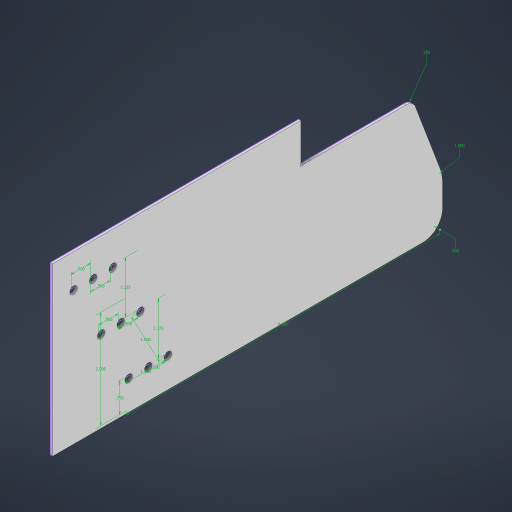
# Autodesk Inventor part: dtplate
Saved by Autodesk Inventor 2024 (Build 280153000, 153)
## iProperties
Created: 2023-11-04
Part Number: dtplate
Material: Generic
Document SubType Name: Modeling
Designer: macbook
Density: 1 g/cm^3
Appearance: Default
Author: macbook
Autodesk Inventor part; units mm, degrees
ref_plane "YZ Plane" through (0, 0, 0) normal (1, 0, 0) x (0, 1, 0)
ref_plane "XZ Plane" through (0, 0, 0) normal (0, 1, 0) x (-1, 0, 0)
ref_plane "XY Plane" through (0, 0, 0) normal (0, 0, 1) x (1, 0, 0)
sketch "Sketch1" plane through (0, 0, 0) normal (1, 0, 0) x (0, 1, 0)
  line L0 (0, -19.05) -> (0, -190.5)
  line L1 (12.7, -203.2) -> (27.1441, -203.2)
  arc A0 (82.55, -117.475) -> (63.5, -95.25) centre (61.8713, -115.9228) ccw
  line L2 (82.55, -117.475) -> (82.55, -179.7494)
  arc A1 (0, -190.5) -> (12.7, -203.2) centre (12.7, -190.5) ccw
  arc A2 (78.4296, -185.6951) -> (82.55, -179.7494) centre (76.2, -179.7494) ccw
  arc A3 (27.1441, -203.2) -> (36.0626, -201.5828) centre (27.1441, -177.8) ccw
  line L3 (78.4296, -185.6951) -> (36.0626, -201.5828)
  line L4 (19.05, 0) -> (19.05, -25.4)
  line L5 (19.05, -25.4) -> (19.05, -12.7)
  line L6 (19.05, -25.4) -> (57.15, -25.4) construction
  line L7 (19.05, -25.4) -> (52.705, -25.4)
  line L8 (52.705, -25.4) -> (52.705, -7.5157)
  line L9 (19.05, -25.4) -> (52.705, -7.5408)
  line L10 (0, -19.05) -> (0, 49.2218)
  line L11 (0, 49.2218) -> (63.5, 49.2218)
  line L12 (52.705, -7.5408) -> (52.705, 5.1592)
  line L13 (52.705, 5.1592) -> (52.705, 17.8592)
  line L14 (52.705, -7.5408) -> (86.36, -7.5408)
  line L15 (52.705, -7.5408) -> (86.36, 10.3184)
  line L16 (86.36, 10.3184) -> (86.36, 23.0184)
  line L17 (86.36, 23.0184) -> (86.36, 35.7184)
  line L18 (86.36, -7.5408) -> (86.36, 10.3184)
  line L19 (63.5, 49.2218) -> (107.8976, 49.2218)
  line L20 (107.8976, 49.2218) -> (107.8976, -111.5493)
  line L21 (107.8976, -111.5493) -> (82.1417, -111.5493)
  point P0 (0, 0)
  point P1 (0, -203.2)
  point P2 (63.5, 0)
  dimension "d0" = 203.2
  dimension "d1" = 63.5
  dimension "d55" = 12.7
  dimension "d56" = 6.35
  dimension "d57" = 25.4
  dimension "d59" = 25.4
  dimension "d60" = 12.7
  dimension "d63" = 33.655
  dimension "d64" = 38.1
  dimension "d65" = 12.7
  dimension "d66" = 12.7
  dimension "d67" = 19.05
  dimension "d68" = 33.655
  dimension "d69" = 12.7
  dimension "d70" = 12.7
  constraints: 44 end point, 9 coincident, 9 point on circle, 7 point on line, 6 vertical, 4 centre point, 4 horizontal, 4 perpendicular, 4 tangent, 1 midpoint
  measures "d0" distance of point (0, 0) point (0, -203.2)
  measures "d1" distance of point (0, 0) point (63.5, 0)
  measures "d55" radius of A1
  measures "d56" radius of A2
  measures "d57" radius of A3
  measures "d59" distance of L4.start L4.end
  measures "d60" distance of L5.start L5.end
  measures "d63" distance of L5.start L7.end
  measures "d64" distance of L5.start L9.end
  measures "d65" distance of L12.start L12.end
  measures "d66" distance of L12.end L13.end
  measures "d67" distance of point (0, 0) L4.start
  measures "d68" distance of L12.start L14.end
  measures "d69" distance of L15.end L16.end
  measures "d70" distance of L16.end L17.end
extrude "Extrusion1" add sketch "Sketch1" along normal blind 1.5875 contours L10 L11 L19 L20 L21 A0 L2 A2 L3 A3 L1 A1 L0 | L9 L8 L7 | L15 L18 L14
hole "Hole3" at (0, 19.05, -25.4) at (0, 19.05, -12.7) at (0, 52.705, -7.5408) at (0, 19.05, 0) at (0, 52.705, 5.1592) at (0, 52.705, 17.8592) at (0, 86.36, 10.3184) at (0, 86.36, 23.0184) at (0, 86.36, 35.7184) direction (1, 0, 0) diameter 4.7625 end through all
body "Solid1"
